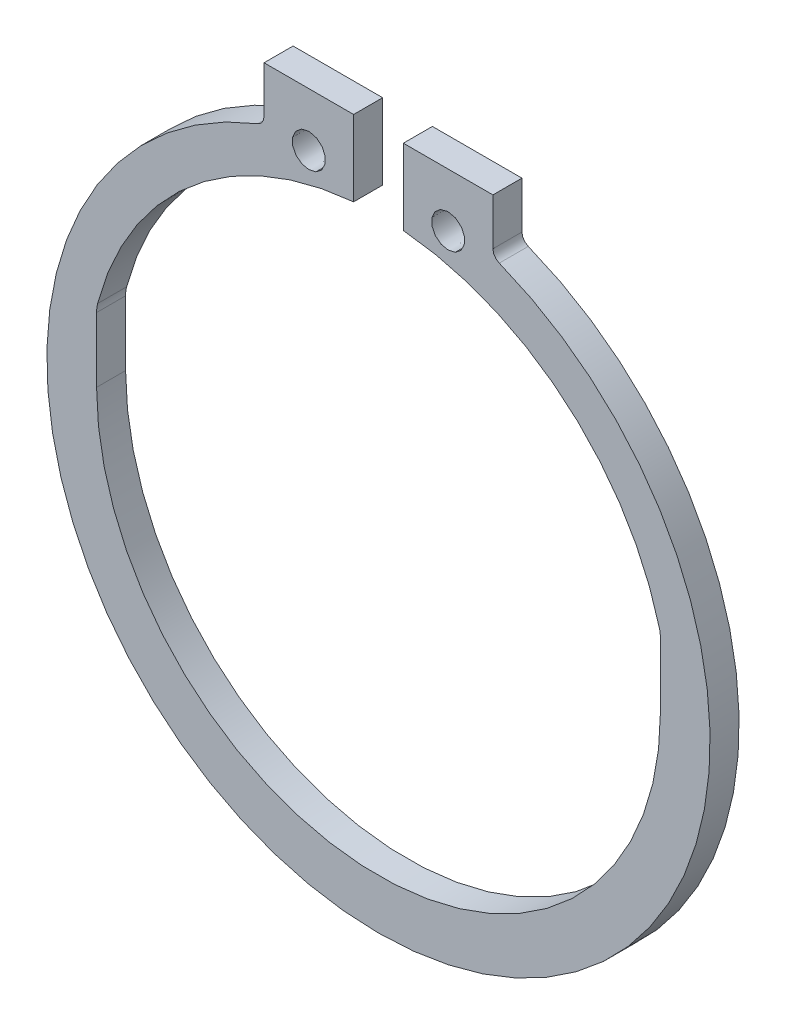
# Autodesk Inventor part: cockring
Saved by Autodesk Inventor 2025 (Build 290162000, 162)
## iProperties
Created: 2025-04-26
Part Number: cockring
Material: Všeobecné
Document SubType Name: Modeling
Designer: jakub
Density: 1 g/cm^3
Appearance: Výchozí
Author: jakub
Autodesk Inventor part; units mm, degrees
ref_plane "YZ Plane" through (0, 0, 0) normal (1, 0, 0) x (0, 1, 0)
ref_plane "XZ Plane" through (0, 0, 0) normal (0, 1, 0) x (-1, 0, 0)
ref_plane "XY Plane" through (0, 0, 0) normal (0, 0, 1) x (1, 0, 0)
sketch "Sketch1" plane through (0, 0, 0) normal (0, 0, 1) x (1, 0, 0)
  circle A0 centre (0, 0) radius 17
  circle A1 centre (0, 0) radius 20
  line L0 (-20, 0) -> (20, 0)
  line L1 (0, 0) -> (0, 20.9298)
  line L2 (0, 20.9298) -> (1.5, 20.9298)
  line L3 (1.5, 20.9298) -> (-1.5, 20.9298)
  line L4 (-1.5, 20.9298) -> (-1.5, 15.3128)
  line L5 (-1.5, 15.3128) -> (1.5, 15.3128)
  line L6 (1.5, 15.3128) -> (1.5, 20.9298)
  line L7 (-20, 0) -> (20, 0)
  point P0 (1.5, 19.9437)
  point P1 (1.5, 16.9337)
  point P2 (-1.5, 16.9337)
  point P3 (-1.5, 19.9437)
  dimension "d0" = 34
  dimension "d1" = 40
  dimension "d2" = 1.5
  dimension "d3" = 3
  constraints: 16 end point, 4 perpendicular, 2 centre point, 2 coincident, 2 horizontal, 2 point on circle, 1 point on line, 1 vertical
  measures "d0" diameter of A0
  measures "d1" diameter of A1
  measures "d2" distance of L1.end L2.end
  measures "d3" distance of L2.end L3.end
extrude "Extrusion1" add sketch "Sketch1" along normal blind 1.75 contours L0 A1 A0 | A0 L6 A1 L0 | L0 A1 L4 A0
sketch "Sketch2" plane through (0, 0, 1.75) normal (0, 0, 1) x (1, 0, 0)
  arc A0 (-1.5, 19.9437) -> (1.5, 19.9437) centre (0, 0) ccw projected
  line L0 (0, -20) -> (0, 22)
  line L1 (1.5, 22) -> (6.9, 22)
  line L2 (6.9, 22) -> (6.9, 18.7721)
  line L3 (1.5, 22) -> (1.5, 19.9437)
  arc A1 (-1.5, 19.9437) -> (1.5, 19.9437) centre (0, 0) ccw
  line L4 (-1.5, 22) -> (-6.9, 22)
  line L5 (-6.9, 22) -> (-6.9, 18.7721)
  line L6 (-1.5, 22) -> (-1.5, 19.9437)
  circle A2 centre (-4.2, 18.7721) radius 1
  circle A3 centre (4.2, 18.7721) radius 1
  point P0 (3.7223, 19.6506)
  point P1 (5.0065, 19.3632)
  point P2 (-5.0065, 19.3632)
  point P3 (-3.7223, 19.6506)
  dimension "d7" = 5.4
  dimension "d8" = 2
  dimension "d9" = 2
  constraints: 14 end point, 5 point on circle, 5 symmetric about line, 3 centre point, 2 vertical, 1 perpendicular, 1 other
  measures "d7" distance of L1.start L1.end
  measures "d8" diameter of A2
  measures "d9" diameter of A3
extrude "Extrusion2" add sketch "Sketch2" against normal blind 1.75 contours A0 A2 L5 L4 L6 | A0 A3 L3 L1 L2
sketch "Sketch3" plane through (0, 0, 0) normal (0, 0, -1) x (-1, 0, 0)
  circle A0 centre (-4.2004, 18.7708) radius 1
  line L0 (0, 22.648) -> (0, 15.9884)
  circle A1 centre (4.2004, 18.7708) radius 1
  point P0 (0, 0)
  dimension "d12" = 2
  constraints: 2 centre point, 2 end point, 1 symmetric about line, 1 vertical, 1 other
  measures "d12" diameter of A0
extrude "Extrusion3" cut sketch "Sketch3" against normal blind 10
fillet "Fillet1" radius 0.6 2 edges at (6.9, 18.7721, 0.875) (-6.9, 18.7721, 0.875)
sketch "Sketch4" plane through (0, 0, 0) normal (0, 0, -1) x (-1, 0, 0)
  circle A0 centre (0, 0) radius 17.5
  line L0 (-17.5, 0) -> (17.5, 0)
  circle A1 centre (0, 0) radius 17
  point P0 (-17, 0)
  point P1 (17, 0)
  dimension "d16" = 35
  constraints: 2 centre point, 2 coincident, 2 end point, 2 point on circle, 1 horizontal
  measures "d16" diameter of A0
extrude "Extrusion4" cut sketch "Sketch4" against normal blind 10 contours L0 A1 A0 picked at (-7.3917, 15.5534)
sketch "Sketch5" plane through (17, 0, 0) normal (0, 1, 0) x (1, 0, 0)
  line L0 (0.5, -1.75) -> (0, -1.75) projected
  line L1 (0, 0) -> (0.5, 0) projected
  line L2 (0.5, -1.75) -> (0, -1.75)
  line L3 (0, -1.75) -> (0, 0)
  line L4 (0, 0) -> (0.5, 0)
  line L5 (0.5, 0) -> (0.5, -1.75)
  point P0 (-17, 0)
  point P1 (0, -1.75)
  constraints: 8 end point, 2 parallel, 1 horizontal, 1 perpendicular
extrude "Extrusion5" add sketch "Sketch5" along normal blind 5
fillet "Fillet2" radius 2 1 edges at (17, 4.1533, 0.875)
sketch "Sketch6" plane through (17, 0, 0) normal (-1, 0, 0) x (0, 0, 1)
  point P0 (0, 0)
mirror "Mirror1" about plane through (0, 0, 0) normal (1, 0, 0) of "Extrusion5"
fillet "Fillet3" radius 2 1 edges at (-17, 4.1533, 0.875)
body "Solid1"
